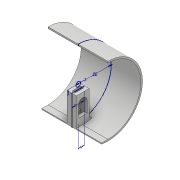
# Autodesk Inventor part: eyes
Saved by Autodesk Inventor 2017 (Build 210142000, 142)
## iProperties
Created: 2018-06-30
Part Number: eyes
Material: Generic
Document SubType Name: Modeling
Designer: mfans
Density: 1 g/cm^3
Appearance: Default
Author: mfans
Autodesk Inventor part; units mm, degrees
ref_plane "YZ Plane" through (0, 0, 0) normal (1, 0, 0) x (0, 1, 0)
ref_plane "XZ Plane" through (0, 0, 0) normal (0, 1, 0) x (-1, 0, 0)
ref_plane "XY Plane" through (0, 0, 0) normal (0, 0, 1) x (1, 0, 0)
sketch "Sketch1" plane through (0, 0, 0) normal (1, 0, 0) x (0, 1, 0)
  arc A0 (0, -22) -> (0, 22) centre (0, 0) ccw
  circle A1 centre (0, 0) radius 1.5
  line L0 (4, -3) -> (-4, -3)
  line L1 (-4, -3) -> (-4, -5.8228)
  line L2 (-4, -5.8228) -> (4, -5.8228)
  line L3 (4, -5.8228) -> (4, -3)
  arc A2 (0, -21) -> (0, 21) centre (0, 0) ccw
  line L4 (-4, -5.8228) -> (-4, -22)
  line L5 (-4, -22) -> (0, -22)
  line L6 (0, -21) -> (-4, -21)
  line L7 (4, -5.8228) -> (4, -20.6155)
  line L8 (0, 21) -> (0, 22)
  line L9 (-4, -21) -> (-4, -22)
  dimension "d0" = 22
  dimension "d1" = 3
  dimension "d2" = 4
  dimension "d3" = 8
  dimension "d4" = 21
  dimension "d5" = 3
  constraints: 20 end point, 5 point on circle, 3 centre point, 3 coincident, 3 perpendicular, 3 vertical, 2 horizontal, 2 parallel, 1 point on line
  measures "d0" radius of A0
  measures "d1" diameter of A1
  measures "d2" distance from line of L3 L5.end
  measures "d3" distance of L1.end L2.end
  measures "d4" radius of A2
  measures "d5" distance from line of point (0, 0) L0
extrude "Extrusion1" add sketch "Sketch1" along normal mid plane 6 contours L4 L2 L7 A2 L6 | L1 L0 L3 L2
sketch "Sketch2" plane through (0, 0, 0) normal (1, 0, 0) x (0, 1, 0)
  arc A0 (0, -21) -> (0, 21) centre (0, 0) ccw projected
  arc A1 (0, -22) -> (0, 22) centre (0, 0) ccw projected
  line L0 (-4, -21) -> (0, -21) projected
  line L1 (-4, -22) -> (0, -22) projected
  line L2 (-4, -21) -> (-4, -22) projected
  line L3 (0, -22) -> (-4, -22)
  line L4 (-4, -3) -> (-4, -21) projected
  line L5 (-4, -22) -> (-4, -21)
  line L6 (-4, -21) -> (0, -21)
  line L7 (0, 22) -> (0, 21)
  constraints: 8 end point, 2 perpendicular, 1 collinear, 1 vertical
extrude "Extrusion2" add sketch "Sketch2" along normal mid plane 38
sketch "Sketch3" plane through (-3, -4, -3) normal (0, 0, 1) x (1, 0, 0)
  line L0 (0, 0) -> (6, 0) projected
  line L1 (6, 8) -> (6, 0) projected
  line L2 (6, 8) -> (0, 8) projected
  line L3 (0, 0) -> (0, 8) projected
  line L4 (4, 1.25) -> (2, 1.25)
  line L5 (2, 1.25) -> (2, 6.75)
  line L6 (2, 6.75) -> (4, 6.75)
  line L7 (4, 6.75) -> (4, 1.25)
  line L8 (4, 1.25) -> (2, 6.75) construction
  line L9 (2, 1.25) -> (4, 6.75) construction
  point P0 (3, 4)
  dimension "d10" = 5.5
  dimension "d11" = 2
  constraints: 12 end point, 2 midpoint, 2 parallel, 1 horizontal, 1 perpendicular
  measures "d10" distance of L4.end L5.end
  measures "d11" distance of L5.end L6.end
extrude "Extrusion3" cut sketch "Sketch3" against normal blind 38 contours L4 L5 L6 L7
sketch "Sketch4" plane through (-19, 0, 0) normal (-1, 0, 0) x (0, 0, 1)
  arc A0 (22, 0) -> (-22, 0) centre (0, 0) ccw projected
  circle A1 centre (0, 0) radius 22
  circle A2 centre (0, 0) radius 26.6183
  constraints: 2 centre point, 2 coincident, 1 concentric
extrude "Extrusion4" cut sketch "Sketch4" along normal through all both and the other way through all
sketch "Sketch5" plane through (-3, 0, 0) normal (-1, 0, 0) x (0, 0, 1)
  line L0 (-3, -4) -> (-3, 4) projected
  line L1 (-3, 4) -> (-20.6155, 4) projected
  arc A0 (-20.6155, 4) -> (-21, 0) centre (0, 0) ccw projected
  line L2 (-21, 0) -> (-21, -4) projected
  line L3 (-21, -4) -> (-3, -4) projected
  line L4 (-3, 2.75) -> (-21.8274, 2.75) projected
  line L5 (-16, -2.75) -> (-6, -2.75)
  line L6 (-6, -2.75) -> (-6, 2.75)
  line L7 (-6, 2.75) -> (-16, 2.75)
  line L8 (-16, 2.75) -> (-16, -2.75)
  line L9 (-16, -2.75) -> (-6, 2.75) construction
  line L10 (-6, -2.75) -> (-16, 2.75) construction
  point P0 (-11, 0)
  dimension "d16" = 10
  dimension "d17" = 3
  constraints: 12 end point, 2 midpoint, 2 parallel, 1 horizontal, 1 perpendicular, 1 point on line
  measures "d16" distance of L5.start L5.end
  measures "d17" distance between parallel lines of L0 L6
extrude "Extrusion5" cut sketch "Sketch5" against normal through all contours L6 L5 L8 L4
chamfer "Chamfer1" distance 2 angle 45 1 edges at (0, 4, -20.6155)
fillet "Fillet1" radius 2.75 4 edges at (-2, 2.75, -6) (2, 2.75, -6) (-2, -2.75, -6) (2, -2.75, -6)
body "Solid1"
